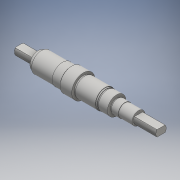
# Autodesk Inventor part: Stator_Axis
Saved by Autodesk Inventor 2016 (Build 200138000, 138)
## iProperties
Created: 2015-11-24
Part Number: Stator_Axis
Material: Générique
Document SubType Name: Modeling
Designer: Cyril
Density: 1 g/cm^3
Appearance: Par défaut
Author: Cyril
Autodesk Inventor part; units mm, degrees
ref_plane "YZ Plane" through (0, 0, 0) normal (1, 0, 0) x (0, 1, 0)
ref_plane "XZ Plane" through (0, 0, 0) normal (0, 1, 0) x (-1, 0, 0)
ref_plane "XY Plane" through (0, 0, 0) normal (0, 0, 1) x (1, 0, 0)
sketch "Esquisse1" plane through (0, 0, 0) normal (0, 0, 1) x (1, 0, 0)
  line L0 (-110, 0) -> (-110, 7)
  line L1 (-110, 7) -> (-109, 8)
  line L2 (-109, 8) -> (-80, 8)
  line L3 (-80, 8) -> (-80, 13)
  line L4 (-80, 13) -> (-75, 13)
  line L5 (-75, 13) -> (-75, 15.5)
  line L6 (-75, 15.5) -> (-42.5, 15.5)
  line L7 (-110, 0) -> (110, 0)
  line L8 (-42.5, 15.5) -> (-42.5, 16)
  line L9 (-42.5, 16) -> (-30, 16)
  arc A0 (-30, 16) -> (-28.25, 16.5) centre (-29.1964, 16.5) ccw
  line L10 (-28.25, 16.5) -> (-28.25, 18)
  line L11 (-28.25, 18) -> (-10.25, 18)
  line L12 (-10.25, 18) -> (-10.25, 14.25)
  line L13 (-10.25, 14.25) -> (-7.75, 14.25)
  line L14 (-7.75, 14.25) -> (-7.75, 15)
  line L15 (-7.75, 15) -> (23.25, 15)
  line L16 (23.25, 15) -> (23.25, 14.25)
  line L17 (23.25, 14.25) -> (25.25, 14.25)
  line L18 (25.25, 14.25) -> (25.25, 13.5)
  line L19 (25.25, 13.5) -> (27.25, 13.5)
  line L20 (27.25, 13.5) -> (27.25, 14.25)
  line L21 (27.25, 14.25) -> (41.25, 14.25)
  line L22 (41.25, 14.25) -> (41.25, 9.5)
  line L23 (41.25, 9.5) -> (43.25, 9.5)
  line L24 (43.25, 9.5) -> (43.25, 10.5)
  line L25 (43.25, 10.5) -> (54.25, 10.5)
  line L26 (54.25, 10.5) -> (54.25, 10)
  line L27 (54.25, 10) -> (75, 10)
  line L28 (75, 10) -> (75, 8)
  line L29 (75, 8) -> (110, 8)
  line L30 (110, 8) -> (110, 0)
  point P0 (0, 0)
  dimension "d0" = 35
  dimension "d1" = 1
  dimension "d2" = 1
  dimension "d3" = 8
  dimension "d4" = 30
  dimension "d5" = 13
  dimension "d6" = 15.5
  dimension "d7" = 16
  dimension "d8" = 32.5
  dimension "d9" = 12.5
  dimension "d10" = 14.25
  dimension "d11" = 0.5
  dimension "d12" = 18
  dimension "d13" = 18
  dimension "d14" = 14.25
  dimension "d15" = 2.5
  dimension "d16" = 75
  dimension "d17" = 15
  dimension "d18" = 31
  dimension "d19" = 2
  dimension "d20" = 2
  dimension "d21" = 14.25
  dimension "d22" = 13.5
  dimension "d23" = 14.25
  dimension "d24" = 14
  dimension "d25" = 9.5
  dimension "d26" = 2
  dimension "d27" = 75
  dimension "d28" = 10.5
  dimension "d29" = 11
  dimension "d30" = 10
  dimension "d31" = 220
  dimension "d32" = 8
  constraints: 62 end point, 15 horizontal, 15 vertical, 2 point on circle, 1 centre point, 1 midpoint, 1 tangent
  measures "d0" distance between parallel lines of L5 L0
  measures "d1" horizontal distance of L0.end L1.end
  measures "d2" horizontal distance of L0.end L1.end
  measures "d3" distance between parallel lines of L7 L2
  measures "d4" distance between parallel lines of L3 L0
  measures "d5" distance between parallel lines of L7 L4
  measures "d6" distance between parallel lines of L7 L6
  measures "d7" distance between parallel lines of L7 L9
  measures "d8" distance of L5.end L6.end
  measures "d9" distance of L8.end L9.end
  measures "d10" distance between parallel lines of L10 L8
  measures "d11" distance from line of L9 A0.centre
  measures "d12" distance between parallel lines of L7 L11
  measures "d13" distance of L10.end L11.end
  measures "d14" distance between parallel lines of L7 L13
  measures "d15" distance of L12.end L13.end
  measures "d16" distance from line of point (0, 0) L5
  measures "d17" distance between parallel lines of L7 L15
  measures "d18" distance of L14.end L15.end
  measures "d19" distance of L16.end L17.end
  measures "d20" distance of L18.end L19.end
  measures "d21" distance between parallel lines of L7 L17
  measures "d22" distance between parallel lines of L7 L19
  measures "d23" distance between parallel lines of L7 L21
  measures "d24" distance of L20.end L21.end
  measures "d25" distance between parallel lines of L7 L23
  measures "d26" distance of L22.end L23.end
  measures "d27" distance from line of point (0, 0) L28
  measures "d28" distance between parallel lines of L7 L25
  measures "d29" distance of L24.end L25.end
  measures "d30" distance between parallel lines of L7 L27
  measures "d31" distance between parallel lines of L30 L0
  measures "d32" distance between parallel lines of L7 L29
revolve "Révolution1" add sketch "Esquisse1" angle 360 about axis through (-110, 0, 0) along (1, 0, 0)
thread "Filetage1" size "M16x1.5" class "6g" standard "ISO Metric profile" full length
sketch "Esquisse2" plane through (-110, 0, 0) normal (-1, 0, 0) x (0, 0, 1)
  circle A0 centre (0, 0) radius 9.5 projected
  line L0 (5, -8.0777) -> (-5, -8.0777)
  line L1 (-5, -8.0777) -> (-5, 8.0777)
  line L2 (-5, 8.0777) -> (5, 8.0777)
  line L3 (5, 8.0777) -> (5, -8.0777)
  line L4 (5, -8.0777) -> (-5, 8.0777) construction
  line L5 (-5, -8.0777) -> (5, 8.0777) construction
  dimension "d34" = 10
  constraints: 12 end point, 2 midpoint, 2 parallel, 1 horizontal, 1 perpendicular, 2 other
  measures "d34" distance of L1.end L2.end
extrude "Extrusion1" cut sketch "Esquisse2" against normal up to surface (30 mm away) contours A0 L3 | L2 A0 | A0 L0 | L1 A0
thread "Filetage4" size "M16x1.5" class "6g" standard "ISO Metric profile" full length
sketch "Esquisse3" plane through (110, 0, 0) normal (1, 0, 0) x (0, 0, -1)
  line L0 (5, -8.6603) -> (-5, -8.6603)
  line L1 (-5, -8.6603) -> (-5, 8.6603)
  line L2 (-5, 8.6603) -> (5, 8.6603)
  line L3 (5, 8.6603) -> (5, -8.6603)
  line L4 (5, -8.6603) -> (-5, 8.6603) construction
  line L5 (-5, -8.6603) -> (5, 8.6603) construction
  circle A0 centre (0, 0) radius 10 projected
  dimension "d45" = 10
  constraints: 12 end point, 2 midpoint, 2 parallel, 1 horizontal, 1 perpendicular, 2 other
  measures "d45" distance of L1.end L2.end
extrude "Extrusion2" cut sketch "Esquisse3" against normal up to surface (35 mm away) contours A0 L0 | L3 A0 | A0 L1 | L2 A0
